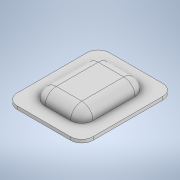
# Autodesk Inventor part: Airpods Pro Base
Saved by Autodesk Inventor 2020 (Build 240168000, 168)
## iProperties
Created: 2020-05-21
Part Number: Airpods Pro Base
Material: Generic
Document SubType Name: Modeling
Designer: maple
Density: 1 g/cm^3
Appearance: Default
Author: maple
Autodesk Inventor part; units mm, degrees
ref_plane "YZ Plane" through (0, 0, 0) normal (1, 0, 0) x (0, 1, 0)
ref_plane "XZ Plane" through (0, 0, 0) normal (0, 1, 0) x (-1, 0, 0)
ref_plane "XY Plane" through (0, 0, 0) normal (0, 0, 1) x (1, 0, 0)
sketch "Sketch1" plane through (0, 0, 0) normal (0, 1, 0) x (-1, 0, 0)
  line L0 (0, 0) -> (-45.2, 0)
  line L1 (-45.2, 0) -> (-45.2, -60.6)
  line L2 (-45.2, -60.6) -> (0, -60.6)
  line L3 (0, -60.6) -> (0, 0)
  dimension "d0" = 45.2
  dimension "d1" = 60.6
  constraints: 8 end point, 2 parallel, 1 horizontal, 1 perpendicular
  measures "d0" distance of L2.end L1.end
  measures "d1" distance of L1.end L0.end
extrude "Extrusion1" add sketch "Sketch1" along normal blind 10.58
fillet "Fillet1" radius 10.58 4 edges at (45.2, 5.29, 0) (45.2, 5.29, -60.6) (0, 5.29, -60.6) (0, 5.29, 0)
fillet "Fillet2" radius 10.58 8 edges at (42.1012, 10.58, -57.5012) (22.6, 10.58, -60.6) (3.0988, 10.58, -57.5012) (0, 10.58, -30.3) (3.0988, 10.58, -3.0988) (22.6, 10.58, 0) (42.1012, 10.58, -3.0988) (45.2, 10.58, -30.3)
sketch "Sketch3" plane through (0, 0, 0) normal (0, -1, 0) x (1, 0, 0)
  line L0 (0, 0) -> (-13, 0)
  line L1 (-13, 0) -> (-13, 13)
  line L2 (-13, 13) -> (0, 13)
  line L3 (0, 13) -> (0, 0)
  line L4 (34.62, -50.02) -> (34.62, -10.58) projected
  line L5 (34.62, -50.02) -> (45.2, -50.02)
  line L6 (45.2, -50.02) -> (45.2, -60.6)
  line L7 (45.2, -60.6) -> (34.62, -60.6)
  line L8 (34.62, -60.6) -> (34.62, -50.02)
  line L9 (45.2, -60.6) -> (58.2, -60.6)
  line L10 (58.2, -60.6) -> (58.2, -73.6)
  line L11 (58.2, -73.6) -> (45.2, -73.6)
  line L12 (45.2, -73.6) -> (45.2, -60.6)
  line L13 (-13, 13) -> (58.2, 13)
  line L14 (58.2, 13) -> (58.2, -73.6)
  line L15 (58.2, -73.6) -> (-13, -73.6)
  line L16 (-13, -73.6) -> (-13, 13)
  dimension "d14" = 13
  dimension "d15" = 13
  dimension "d16" = 13
  dimension "d17" = 13
  constraints: 32 end point, 8 parallel, 4 horizontal, 4 perpendicular
  measures "d14" distance of L1.end L2.end
  measures "d15" distance of L0.end L1.end
  measures "d16" distance of L10.end L11.end
  measures "d17" distance of L9.end L10.end
extrude "Extrusion3" add sketch "Sketch3" along normal blind 3 contours L7 L8 L5 L6 | L3 L13 L14 L9 L12 L15 L16 L0 | L0 L1 L2 L3 | L12 L9 L10 L11
fillet "Fillet4" radius 10.58 4 edges at (-13, -1.5, 13) (-13, -1.5, -73.6) (58.2, -1.5, -73.6) (58.2, -1.5, 13)
body "Solid1"
